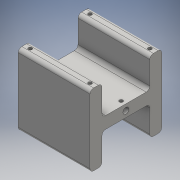
# Autodesk Inventor part: 60x60Idler
Saved by Autodesk Inventor 2016 (Build 200138000, 138)
## iProperties
Created: 2016-05-22
Part Number: 60x60Idler
Material: Generic
Document SubType Name: Modeling
Designer: Kurtis
Density: 1 g/cm^3
Appearance: Default
Author: Kurtis
Autodesk Inventor part; units mm, degrees
ref_plane "YZ Plane" through (0, 0, 0) normal (1, 0, 0) x (0, 1, 0)
ref_plane "XZ Plane" through (0, 0, 0) normal (0, 1, 0) x (-1, 0, 0)
ref_plane "XY Plane" through (0, 0, 0) normal (0, 0, 1) x (1, 0, 0)
sketch "Sketch1" plane through (0, 0, 0) normal (0, 0, 1) x (1, 0, 0)
  line L0 (-30, -30) -> (30, -30)
  line L1 (30, -30) -> (30, 30)
  line L2 (30, 30) -> (-30, 30)
  line L3 (-30, 30) -> (-30, -30)
  line L4 (-30, -30) -> (30, 30) construction
  line L5 (30, -30) -> (-30, 30) construction
  line L6 (30, 30) -> (25, 30) construction
  line L7 (25, 30) -> (25, 25) construction
  line L8 (-30, 30) -> (-25, 30) construction
  line L9 (-25, 30) -> (-25, 25) construction
  line L10 (-30, -30) -> (-30, -25) construction
  line L11 (-30, -25) -> (-25, -25) construction
  line L12 (30, -30) -> (30, -25) construction
  line L13 (30, -25) -> (25, -25) construction
  circle A0 centre (-25, 25) radius 1.5
  circle A1 centre (25, 25) radius 1.5
  circle A2 centre (25, -25) radius 1.5
  circle A3 centre (-25, -25) radius 1.5
  point P0 (0, 0)
  dimension "d0" = 60
  dimension "d1" = 60
  dimension "d2" = 5
  dimension "d3" = 5
  dimension "d4" = 5
  dimension "d5" = 5
  dimension "d6" = 5
  dimension "d7" = 5
  dimension "d8" = 5
  dimension "d9" = 5
  dimension "d10" = 3
  dimension "d11" = 3
  dimension "d12" = 3
  dimension "d13" = 3
  constraints: 28 end point, 8 point on line, 4 centre point, 4 coincident, 2 midpoint, 2 parallel, 1 horizontal, 1 perpendicular
  measures "d0" distance of L2.end L1.end
  measures "d1" distance of L1.end L0.end
  measures "d2" distance of L1.end L6.end
  measures "d3" distance of L6.end L7.end
  measures "d4" distance of L2.end L8.end
  measures "d5" distance of L8.end L9.end
  measures "d6" distance of L0.start L10.end
  measures "d7" distance of L10.end L11.end
  measures "d8" distance of L0.end L12.end
  measures "d9" distance of L12.end L13.end
  measures "d10" diameter of A0
  measures "d11" diameter of A1
  measures "d12" diameter of A2
  measures "d13" diameter of A3
extrude "Block" add sketch "Sketch1" along normal blind 60
sketch "Sketch2" plane through (30, -30, 0) normal (1, 0, 0) x (0, 0, -1)
  line L0 (0, 0) -> (0, 60) construction
  line L1 (-60, 0) -> (0, 60) construction
  circle A0 centre (-30, 30) radius 2.5
  point P0 (0, 30)
  dimension "d17" = 5
  constraints: 2 end point, 1 centre point, 1 midpoint
  measures "d17" diameter of A0
extrude "Motor Mount" cut sketch "Sketch2" against normal blind 60
sketch "Sketch3" plane through (30, -30, 0) normal (1, 0, 0) x (0, 0, -1)
  line L0 (0, 60) -> (-60, 60) construction
  line L1 (-60, 60) -> (-60, 50) construction
  line L2 (-60, 60) -> (-60, 0) construction
  line L3 (-60, 50) -> (0, 50) construction
  line L4 (0, 60) -> (0, 0) construction
  line L5 (-60, 0) -> (-60, 10) construction
  line L6 (-60, 10) -> (0, 10) construction
  circle A0 centre (-30, 30) radius 2.5 construction
  line L7 (-30, 30) -> (-25, 30) construction
  line L8 (-30, 30) -> (-35, 30) construction
  line L9 (-35, 30) -> (-35, 10) construction
  line L10 (-25, 30) -> (-25, 10) construction
  line L11 (-25, 30) -> (-25, 50) construction
  line L12 (-35, 30) -> (-35, 50) construction
  line L13 (-60, 50) -> (-35, 50)
  line L14 (-35, 10) -> (-60, 10)
  line L15 (-35, 10) -> (-35, 50)
  line L16 (-25, 50) -> (-25, 10)
  line L17 (0, 10) -> (-25, 10)
  line L18 (-25, 50) -> (0, 50)
  line L19 (0, 50) -> (0, 10)
  line L20 (-60, 10) -> (-60, 50)
  point P0 (0, 30)
  dimension "d20" = 10
  dimension "d21" = 10
  dimension "d22" = 5
  dimension "d23" = 5
  constraints: 36 end point, 10 point on line, 8 perpendicular, 4 collinear, 2 horizontal
  measures "d20" distance of L0.end L1.end
  measures "d21" distance of L2.end L5.end
  measures "d22" distance of L7.start L7.end
  measures "d23" distance of L7.start L8.end
extrude "Plastic Savings" cut sketch "Sketch3" against normal blind 60
fillet "Fillets FTW" radius 3 12 edges at (0, -30, 60) (0, -20, 60) (0, 30, 60) (0, 20, 60) (0, 20, 35) (0, -20, 35) (0, -20, 0) (0, -30, 0) (0, -20, 25) (0, 20, 25) (0, 30, 0) (0, 20, 0)
sketch "Sketch4" plane through (30, -17, 35) normal (0, 0, 1) x (1, 0, 0)
  line L0 (0, 19.5) -> (0, 14.5) construction
  line L1 (0, 17) -> (-4, 17) construction
  circle A0 centre (-4, 17) radius 1.5
  point P0 (-30, 17)
  dimension "d27" = 4
  dimension "d28" = 3
  constraints: 2 end point, 1 centre point, 1 coincident, 1 horizontal, 1 midpoint
  measures "d27" distance of L1.start L1.end
  measures "d28" diameter of A0
extrude "Axle Lock" cut sketch "Sketch4" against normal blind 3.75
body "Solid1"
